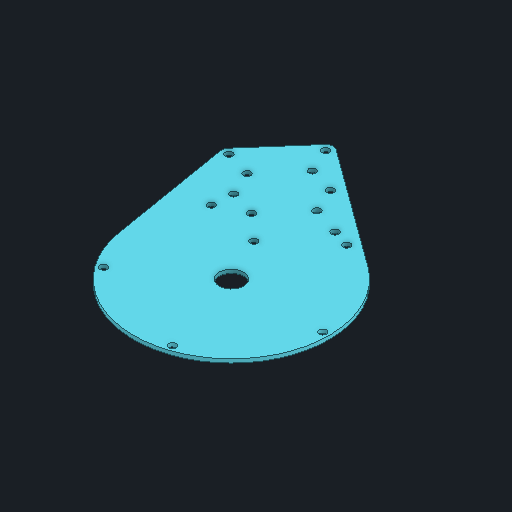
# Autodesk Inventor part: femur_motor_steel
Saved by Autodesk Inventor 2026 (Build 300175000, 175)
## iProperties
Created: 2026-04-24
Part Number: femur_motor_steel
Material: Сталь
Document SubType Name: Modeling
Designer: user
Density: 7.85 g/cm^3
Appearance: Серо-синий
Mass: 592.17 g
Surface Area: 531.53 cm^2
Volume: 75.4357 cm^3
Author: user
Autodesk Inventor part; units mm, degrees
ref_plane "YZ Plane" through (0, 0, 0) normal (1, 0, 0) x (0, 1, 0)
ref_plane "XZ Plane" through (0, 0, 0) normal (0, 1, 0) x (-1, 0, 0)
ref_plane "XY Plane" through (0, 0, 0) normal (0, 0, 1) x (1, 0, 0)
sketch "Эскиз1" plane through (0, 0, 0) normal (0, 1, 0) x (-1, 0, 0)
  circle A0 centre (-168.9344, 188.7011) radius 10 projected
  circle A1 centre (-151.3339, 152.7042) radius 3.05 projected
  circle A2 centre (-130.5866, 133.819) radius 3.05 projected
  circle A3 centre (-109.5427, 127.4971) radius 3.05 projected
  circle A4 centre (-100.4838, 107.4784) radius 3.05 projected
  circle A5 centre (-79.44, 101.1565) radius 3.05 projected
  circle A6 centre (-116.3826, 58.9374) radius 3.05 projected
  circle A7 centre (-125.4415, 78.9561) radius 3.05 projected
  circle A8 centre (-146.4853, 85.278) radius 3.05 projected
  circle A9 centre (-155.5442, 105.2966) radius 3.05 projected
  circle A10 centre (-178.0556, 112.9027) radius 3.05 projected
  circle A11 centre (-168.9344, 188.7011) radius 75 construction
  circle A12 centre (-108.2116, 232.7209) radius 3.05
  circle A13 centre (-192.0353, 260.0548) radius 3.05
  circle A14 centre (-243.9343, 188.7803) radius 3.05
  circle A15 centre (-192.186, 117.3964) radius 3.05
  circle A16 centre (-108.3047, 144.5532) radius 3.05
  arc A17 (-90.0208, 201.8409) -> (-216.0616, 124.0558) centre (-168.9344, 188.7011) ccw
  arc A18 (-74.8493, 97.1396) -> (-73.4228, 102.1585) centre (-79.44, 101.1565) ccw
  arc A19 (-119.976, 54.0082) -> (-111.7919, 54.9205) centre (-116.3826, 58.9374) ccw
  line L0 (-90.0208, 201.8409) -> (-73.4228, 102.1585)
  line L1 (-216.0616, 124.0558) -> (-119.976, 54.0082)
  line L2 (-111.7919, 54.9205) -> (-74.8493, 97.1396)
  point P0 (0, 0)
  dimension "d4" = 150
  dimension "d5" = 6.1
  dimension "d8" = 360
  dimension "d10" = 160
  dimension "d11" = 12.2
  dimension "d12" = 12.2
  constraints: 8 centre point, 6 end point, 6 point on circle, 6 tangent, 4 coincident, 14 other
  measures "d5" diameter of A12
  measures "d10" diameter of A17
  measures "d11" diameter of A18
  measures "d12" diameter of A19
extrude "Выдавливание1" add sketch "Эскиз1" along normal blind 3
equation "\"d5\" = d_main_screw_holes"
equation "\"d11\" = 2 * d_main_screw_holes"
equation "\"d12\" = 2 * d_main_screw_holes"
equation "\"d2\" = thickness_steel"
equation "\"tolerance_plazma\" = 0.1"
equation "\"thickness_steel\" = 3"
equation "\"d_main_screw_holes\" = 6.1"
equation "\"d_main_shaft\" = 16"
equation "\"thickness_profile_tibea\" = 4"
equation "\"thickness_profile_femur\" = 3"
equation "\"width_shaft_shift\" = 35"
equation "\"width_flattened_surface\" = 12"
